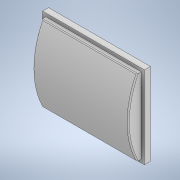
# Autodesk Inventor part: MainHousing_Screen Acrylic
Saved by Autodesk Inventor 2021 (Build 250183000, 183)
## iProperties
Created: 2021-04-29
Part Number: MainHousing_Screen Acrylic
Material: Generic
Document SubType Name: Modeling
Designer: trent
Density: 1 g/cm^3
Appearance: Default
Author: trent
Autodesk Inventor part; units mm, degrees
ref_plane "YZ Plane" through (0, 0, 0) normal (1, 0, 0) x (0, 1, 0)
ref_plane "XZ Plane" through (0, 0, 0) normal (0, 1, 0) x (-1, 0, 0)
sketch "Sketch1" plane through (0, 0, 0) normal (0, 0, 1) x (1, 0, 0)
  line L0 (0, 0) -> (94, 0)
  line L1 (94, 0) -> (94, 76)
  line L2 (94, 76) -> (0, 76)
  line L3 (0, 76) -> (0, 0)
  line L4 (4.75, 10.5) -> (89.25, 10.5)
  line L5 (89.25, 10.5) -> (89.25, 65.5)
  line L6 (89.25, 65.5) -> (4.75, 65.5)
  line L7 (4.75, 65.5) -> (4.75, 10.5)
  dimension "d0" = 84.5
  dimension "d1" = 55
  dimension "d2" = 76
  dimension "d3" = 94
  dimension "d4" = 10.5
  dimension "d5" = 4.75
  dimension "d6" = 4.75
  dimension "d7" = 10.5
  constraints: 16 end point, 4 parallel, 2 horizontal, 2 perpendicular
  measures "d0" distance of L5.end L6.end
  measures "d1" distance of L4.end L5.end
  measures "d2" distance of L0.end L1.end
  measures "d3" distance of L1.end L2.end
  measures "d4" distance between parallel lines of L2 L6
  measures "d5" distance between parallel lines of L3 L7
  measures "d6" distance between parallel lines of L1 L5
  measures "d7" distance between parallel lines of L0 L4
extrude "Extrusion1" add sketch "Sketch1" along normal blind 17.5 contours L3 L2 L1 L0 | L7 L6 L5 L4
ref_plane "Work Plane1" through (0, 0, 18) normal (0, 0, -1) x (-1, 0, 0)
sketch "Sketch3" plane through (0, 0, 18) normal (0, 0, -1) x (-1, 0, 0)
  line L0 (0, 0) -> (-94, 0) projected
  line L1 (0, 76) -> (-3, 76)
  line L2 (-3, 76) -> (-3, 0)
  line L3 (-3, 0) -> (0, 0)
  line L4 (0, 0) -> (0, 76)
  line L5 (-94, 0) -> (-91, 0)
  line L6 (-91, 0) -> (-91, 76)
  line L7 (-91, 76) -> (-94, 76)
  line L8 (-94, 76) -> (-94, 0)
  line L9 (-94, 76) -> (0, 76) projected
  dimension "d16" = 3
  dimension "d17" = 3
  dimension "d32" = 0
  constraints: 16 end point, 4 parallel, 2 horizontal, 2 perpendicular, 1 point on line
  measures "d16" distance of L1.start L1.end
  measures "d17" distance of L6.end L7.end
  measures "d32" distance between parallel lines of L9 L7
extrude "Extrusion3" cut sketch "Sketch3" along normal blind 12.5 contours L0 L2 L1 L4 | L0 L8 L7 L6
sketch "Sketch4" plane through (0, 0, 18) normal (0, 0, -1) x (-1, 0, 0)
  line L0 (0, 76) -> (0, 0) projected
  line L1 (-94, 76) -> (-94, 0) projected
  line L2 (0, 76) -> (-94, 76)
  line L3 (-94, 76) -> (-94, 73)
  line L4 (-94, 73) -> (0, 73)
  line L5 (0, 73) -> (0, 76)
  line L6 (-104.5, 0) -> (0, 0) projected
  line L7 (0, 0) -> (-94, 0)
  line L8 (-94, 0) -> (-94, 3)
  line L9 (-94, 3) -> (0, 3)
  line L10 (0, 3) -> (0, 0)
  point P0 (-104.5, 75.9892)
  point P1 (-104.5, 3.0108)
  point P2 (0, 3)
  point P3 (-94, 3)
  point P4 (-94, 3)
  point P5 (-94, 0)
  point P6 (-104.5, 75.9892)
  point P7 (-95, 6)
  dimension "d20" = 3
  dimension "d21" = 3
  constraints: 16 end point, 4 parallel, 2 horizontal, 2 perpendicular, 1 point on line, 2 other
  measures "d20" distance of L2.end L3.end
  measures "d21" distance of L7.end L8.end
extrude "Extrusion4" cut sketch "Sketch4" along normal blind 12.5 contours L0 L4 L1 L2 | L0 L6 L1 L9
sketch "Sketch5" plane through (94, 0, 0) normal (1, 0, 0) x (0, 0, -1)
  line L0 (-17.5, 3) -> (-17.5, 73) projected
  line L1 (0, 76) -> (-5.5, 76) projected
  line L2 (0, 0) -> (-5.5, 0) projected
  arc A0 (-7.5, 76) -> (-7.5, 0) centre (59.7, 38) ccw
  line L3 (0, 0) -> (0, 76) projected
  line L4 (-17.5, 38) -> (-17.5, 3)
  line L5 (-17.5, 3) -> (-5.5, 3) projected
  line L6 (-9.1102, 3) -> (-17.5, 3)
  line L7 (-5.5, 73) -> (-17.5, 73) projected
  line L8 (-9.1102, 73) -> (-17.5, 73)
  line L9 (-17.5, 73) -> (-17.5, 38)
  point P0 (-15, 3)
  point P1 (-15, 73)
  point P2 (-15, 73)
  point P3 (-15, 3)
  dimension "d24" = 38
  dimension "d25" = 38
  dimension "d26" = 7.5
  dimension "d27" = 7.5
  constraints: 8 end point, 5 point on circle, 4 point on line, 1 centre point, 1 collinear, 1 horizontal, 1 midpoint, 1 vertical
  measures "d24" distance from line of L1 L4.start
  measures "d25" distance from line of L2 L4.start
  measures "d26" distance from line of L3 A0.start
  measures "d27" distance from line of L3 A0.end
extrude "Extrusion5" cut sketch "Sketch5" against normal through all
fillet "Fillet1" radius 1 4 edges at (47, 73, 9.1102) (91, 38, 17.5) (3, 38, 17.5) (47, 3, 9.1102)
equation "\"d17\" = d16"
equation "\"d21\" = d20"
equation "\"d27\" = d26"
body "Solid1"
